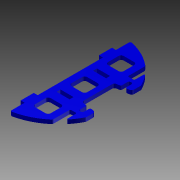
# Autodesk Inventor part: OpenROV 2.3 Dev EBoard Plug Mount
Saved by Autodesk Inventor 2012 (Build 160160000, 160)
## iProperties
Created: 2011-12-20
Part Number: OpenROV 2.3 Dev EBoard Plug Mount
Document SubType Name: Modeling
Designer: user
Density: 1 g/cm^3
Material: Default
Author: user
Autodesk Inventor part; units mm, degrees
ref_plane "YZ Plane" through (0, 0, 0) normal (1, 0, 0) x (0, 1, 0)
ref_plane "XZ Plane" through (0, 0, 0) normal (0, 1, 0) x (-1, 0, 0)
ref_plane "XY Plane" through (0, 0, 0) normal (0, 0, 1) x (1, 0, 0)
sketch "Sketch1" plane through (0, 0, 0) normal (0, 0, 1) x (1, 0, 0)
  line L0 (1.7529, 25) -> (4.7529, 25)
  line L1 (4.7529, 35) -> (1.7529, 35)
  line L2 (1.7529, 35) -> (1.7529, 25)
  line L3 (1.7529, -25) -> (4.7529, -25)
  line L4 (4.7529, -35) -> (1.7529, -35)
  line L5 (1.7529, -35) -> (1.7529, -25)
  line L6 (26.0029, -10.7424) -> (26.0029, 10.7264)
  line L7 (38.0029, -20.6235) -> (38.0029, -15.7736)
  line L8 (38.0029, 15.7576) -> (38.0029, 20.6075)
  line L9 (36.251, 13.773) -> (34.6269, 13.57)
  line L10 (29.6269, 12.945) -> (27.7548, 12.711)
  line L11 (36.251, -13.789) -> (34.6271, -13.586)
  line L12 (29.6269, -12.961) -> (27.7548, -12.727)
  arc A0 (26.0029, -10.7424) -> (27.7548, -12.727) centre (28.0029, -10.7424) ccw
  arc A1 (27.7548, 12.711) -> (26.0029, 10.7264) centre (28.0029, 10.7264) ccw
  arc A2 (38.0029, -15.7736) -> (36.251, -13.789) centre (36.0029, -15.7736) ccw
  arc A3 (36.251, 13.773) -> (38.0029, 15.7576) centre (36.0029, 15.7576) ccw
  arc A4 (30.5029, -13.9533) -> (29.6269, -12.961) centre (29.5029, -13.9533) ccw
  arc A5 (34.6271, -13.586) -> (33.5031, -14.5783) centre (34.5031, -14.5783) ccw
  arc A6 (33.5029, 14.5623) -> (34.6269, 13.57) centre (34.5029, 14.5623) ccw
  arc A7 (29.6269, 12.945) -> (30.5029, 13.9373) centre (29.5029, 13.9373) ccw
  arc A8 (38.0029, 20.6075) -> (37.7807, 21.5238) centre (36.0029, 20.6075) ccw
  arc A9 (37.7807, -21.5398) -> (38.0029, -20.6235) centre (36.0029, -20.6235) ccw
  line L13 (4.7529, -35) -> (4.7529, -44.9628)
  line L14 (4.7529, 35) -> (4.7529, 44.9468)
  line L15 (4.7529, 25) -> (4.7529, -25)
  line L16 (9.7529, -15.508) -> (19.7529, -15.508)
  line L17 (19.7529, -15.508) -> (19.7529, -12.508)
  line L18 (19.7529, -12.508) -> (9.7529, -12.508)
  line L19 (9.7529, -12.508) -> (9.7529, -15.508)
  line L20 (9.7529, 12.492) -> (19.7529, 12.492)
  line L21 (19.7529, 12.492) -> (19.7529, 15.492)
  line L22 (19.7529, 15.492) -> (9.7529, 15.492)
  line L23 (9.7529, 15.492) -> (9.7529, 12.492)
  arc A10 (4.7529, -44.9628) -> (5.9649, -45.9401) centre (5.7529, -44.9628) ccw
  arc A11 (5.9649, 45.9241) -> (4.7529, 44.9468) centre (5.7529, 44.9468) ccw
  line L24 (19.7529, -6.008) -> (11.7529, -6.008)
  line L25 (9.7529, -4.008) -> (9.7529, 3.992)
  line L26 (11.7529, 5.992) -> (19.7529, 5.992)
  line L27 (21.7529, 3.992) -> (21.7529, -4.008)
  line L28 (11.7529, 21.992) -> (19.7529, 21.992)
  line L29 (21.7529, 23.992) -> (21.7529, 31.992)
  line L30 (19.7529, 33.992) -> (11.7529, 33.992)
  line L31 (9.7529, 31.992) -> (9.7529, 23.992)
  line L32 (11.7529, -22.008) -> (19.7529, -22.008)
  line L33 (21.7529, -24.008) -> (21.7529, -32.008)
  line L34 (19.7529, -34.008) -> (11.7529, -34.008)
  line L35 (9.7529, -32.008) -> (9.7529, -24.008)
  arc A12 (11.7529, 5.992) -> (9.7529, 3.992) centre (11.7529, 3.992) ccw
  arc A13 (21.7529, 3.992) -> (19.7529, 5.992) centre (19.7529, 3.992) ccw
  arc A14 (19.7529, -6.008) -> (21.7529, -4.008) centre (19.7529, -4.008) ccw
  arc A15 (9.7529, -4.008) -> (11.7529, -6.008) centre (11.7529, -4.008) ccw
  arc A16 (11.7529, -22.008) -> (9.7529, -24.008) centre (11.7529, -24.008) ccw
  arc A17 (21.7529, -24.008) -> (19.7529, -22.008) centre (19.7529, -24.008) ccw
  arc A18 (19.7529, -34.008) -> (21.7529, -32.008) centre (19.7529, -32.008) ccw
  arc A19 (9.7529, -32.008) -> (11.7529, -34.008) centre (11.7529, -32.008) ccw
  arc A20 (11.7529, 33.992) -> (9.7529, 31.992) centre (11.7529, 31.992) ccw
  arc A21 (21.7529, 31.992) -> (19.7529, 33.992) centre (19.7529, 31.992) ccw
  arc A22 (19.7529, 21.992) -> (21.7529, 23.992) centre (19.7529, 23.992) ccw
  arc A23 (9.7529, 23.992) -> (11.7529, 21.992) centre (11.7529, 23.992) ccw
  line L36 (31.7529, 29.1156) -> (31.7529, 22.992)
  line L37 (30.7529, 21.992) -> (27.7529, 21.992)
  line L38 (26.7529, 22.992) -> (26.7529, 34.6104)
  arc A24 (37.7807, 21.5238) -> (32.6427, 29.4288) centre (-3.9971, -0.008) ccw
  arc A25 (26.0307, 36.149) -> (5.9649, 45.9241) centre (-3.9971, -0.008) ccw
  line L39 (27.7529, -22.008) -> (30.7529, -22.008)
  line L40 (31.7529, -23.008) -> (31.7529, -29.1317)
  line L41 (26.7529, -34.6265) -> (26.7529, -23.008)
  arc A26 (5.9649, -45.9401) -> (26.0307, -36.1651) centre (-3.9971, -0.008) ccw
  arc A27 (32.6427, -29.4448) -> (37.7807, -21.5398) centre (-3.9971, -0.008) ccw
  arc A28 (32.6427, 29.4288) -> (31.7529, 29.1156) centre (32.2529, 29.1156) ccw
  arc A29 (31.7529, -29.1317) -> (32.6427, -29.4448) centre (32.2529, -29.1317) ccw
  arc A30 (26.0307, -36.1651) -> (26.7529, -34.6265) centre (24.7529, -34.6265) ccw
  arc A31 (26.7529, 34.6104) -> (26.0307, 36.149) centre (24.7529, 34.6104) ccw
  arc A32 (30.7529, 21.992) -> (31.7529, 22.992) centre (30.7529, 22.992) ccw
  arc A33 (26.7529, 22.992) -> (27.7529, 21.992) centre (27.7529, 22.992) ccw
  arc A34 (31.7529, -23.008) -> (30.7529, -22.008) centre (30.7529, -23.008) ccw
  arc A35 (27.7529, -22.008) -> (26.7529, -23.008) centre (27.7529, -23.008) ccw
  arc A36 (30.5029, -17.9841) -> (33.5031, -18.008) centre (32.0029, -18.008) ccw
  arc A37 (33.5029, 17.992) -> (30.5029, 17.992) centre (32.0029, 17.992) ccw
  line L42 (30.5029, 17.992) -> (30.5029, 13.9373)
  line L43 (33.5029, 17.992) -> (33.5029, 14.5623)
  line L44 (30.5029, -18.032) -> (30.5029, -13.9533)
  line L45 (33.5031, -18.008) -> (33.5031, -14.5783)
  point P0 (4.7529, -46.1863)
  point P1 (4.7529, 46.1703)
  point P2 (38.0029, -21.103)
  point P3 (38.0029, 21.087)
  point P4 (38.0029, -14.008)
  point P5 (38.0029, 13.992)
  point P6 (26.0029, -12.508)
  point P7 (9.7529, 5.992)
  point P8 (9.7529, -6.008)
  point P9 (21.7529, 5.992)
  point P10 (21.7529, 33.992)
  point P11 (21.7529, 21.992)
  point P12 (9.7529, 33.992)
  point P13 (21.7529, -34.008)
  point P14 (21.7529, -22.008)
  point P15 (9.7529, -34.008)
  point P16 (26.7529, 35.5369)
  point P17 (31.7529, 30.5033)
  point P18 (26.7529, -22.008)
  point P19 (26.7529, -35.5529)
  point P20 (31.7529, -30.5193)
  dimension "d13" = 10
  dimension "d17" = 10
  dimension "d70" = 3
  dimension "d72" = 3
  dimension "d88" = 28
  dimension "d90" = 1.5
  dimension "d92" = 14
  dimension "d99" = 2
  dimension "d100" = 2
  dimension "d101" = 1
  dimension "d102" = 2
  dimension "d105" = 10
  dimension "d106" = 3
  dimension "d107" = 10
  dimension "d108" = 3
  dimension "d109" = 5
  dimension "d110" = 5
  dimension "d111" = 25
  dimension "d112" = 12.5
  dimension "d115" = 1
  dimension "d117" = 8.75
  dimension "d118" = 12
  dimension "d119" = 12
  dimension "d120" = 5
  dimension "d121" = 6.5
  dimension "d123" = 5
  dimension "d126" = 6.5
  dimension "d127" = 12
  dimension "d128" = 12
  dimension "d129" = 6.5
  dimension "d130" = 12
  dimension "d131" = 12
  dimension "d132" = 2
  dimension "d135" = 5
  dimension "d136" = 5
  dimension "d137" = 5
  dimension "d138" = 6.5
  dimension "d139" = 5
  dimension "d140" = 5
  dimension "d141" = 0.5
  dimension "d142" = 2
  dimension "d143" = 1
  dimension "d144" = 3
  dimension "d147" = 4
  dimension "d148" = 4
  constraints: 92 end point, 81 point on circle, 63 tangent, 38 centre point, 36 point on line, 23 equal radius, 18 parallel, 8 horizontal, 6 perpendicular, 1 collinear
  measures "d13" distance of L1.end L0.start
  measures "d17" distance of L4.end L3.start
  measures "d70" distance of L1.start L1.end
  measures "d72" distance of L4.start L4.end
  measures "d88" distance of point (38.003, 13.992) point (38.003, -14.008)
  measures "d90" vertical distance of point (26.003, -12.508) point (38.003, -14.008)
  measures "d92" vertical distance of A24.centre point (38.003, -14.008)
  measures "d99" radius of A0
  measures "d100" radius of A2
  measures "d101" radius of A4
  measures "d102" radius of A8
  measures "d105" distance of L16.start L16.end
  measures "d106" distance of L18.end L16.start
  measures "d107" distance of L21.end L22.end
  measures "d108" distance of L22.end L20.start
  measures "d109" distance between parallel lines of L15 L23
  measures "d110" distance between parallel lines of L15 L19
  measures "d111" distance between parallel lines of L20 L18
  measures "d112" distance from line of L20 A24.centre
  measures "d115" radius of A10
  measures "d117" distance from line of A24.centre L15
  measures "d118" distance of point (9.753, 5.992) point (21.753, 5.992)
  measures "d119" distance of point (9.753, -6.008) point (9.753, 5.992)
  measures "d120" distance between parallel lines of L15 L25
  measures "d121" distance between parallel lines of L20 L26
  measures "d123" distance between parallel lines of L15 L35
  measures "d126" distance between parallel lines of L22 L28
  measures "d127" distance of point (21.753, 21.992) point (21.753, 33.992)
  measures "d128" distance of point (21.753, 33.992) point (9.753, 33.992)
  measures "d129" distance between parallel lines of L32 L16
  measures "d130" distance of point (21.753, -22.008) point (21.753, -34.008)
  measures "d131" distance of point (21.753, -34.008) point (9.753, -34.008)
  measures "d132" radius of A12
  measures "d135" distance between parallel lines of L29 L38
  measures "d136" distance between parallel lines of L15 L31
  measures "d137" distance between parallel lines of L38 L36
  measures "d138" distance between parallel lines of L22 L37
  measures "d139" distance between parallel lines of L33 L41
  measures "d140" distance between parallel lines of L41 L40
  measures "d141" radius of A28
  measures "d142" radius of A30
  measures "d143" radius of A32
  measures "d144" diameter of A37
  measures "d147" distance from line of L39 A36.centre
  measures "d148" distance from line of A37.centre L37
extrude "Extrusion8" add sketch "Sketch1" along normal blind 3
body "Solid8"
